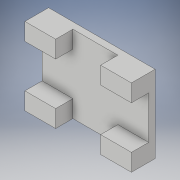
# Autodesk Inventor part: Temporary Guide
Saved by Autodesk Inventor 2018 (Build 220112000, 112)
## iProperties
Created: 2019-01-11
Part Number: Temporary Guide
Material: Generic
Document SubType Name: Modeling
Designer: s-2512711
Density: 1 g/cm^3
Appearance: Default
Author: s-2512711
Autodesk Inventor part; units mm, degrees
ref_plane "YZ Plane" through (0, 0, 0) normal (1, 0, 0) x (0, 1, 0)
ref_plane "XZ Plane" through (0, 0, 0) normal (0, 1, 0) x (-1, 0, 0)
ref_plane "XY Plane" through (0, 0, 0) normal (0, 0, 1) x (1, 0, 0)
sketch "Sketch1" plane through (0, 0, 0) normal (0, 0, 1) x (1, 0, 0)
  line L0 (0, 0) -> (100.33, 0)
  line L1 (100.33, 0) -> (100.33, 72.898)
  line L2 (100.33, 72.898) -> (0, 72.898)
  line L3 (0, 72.898) -> (0, 0)
  dimension "d0" = 100.33
  dimension "d1" = 72.898
  constraints: 8 end point, 2 parallel, 1 horizontal, 1 perpendicular
  measures "d0" distance of L2.end L1.end
  measures "d1" distance of L1.end L0.end
extrude "Extrusion1" add sketch "Sketch1" along normal blind 6.096
sketch "Sketch2" plane through (0, 0, 6.096) normal (0, 0, 1) x (1, 0, 0)
  line L0 (100.33, 72.898) -> (0, 72.898) projected
  line L1 (0, 72.898) -> (28.956, 72.898)
  line L2 (28.956, 72.898) -> (28.956, 56.642)
  line L3 (28.956, 56.642) -> (0, 56.642)
  line L4 (0, 56.642) -> (0, 72.898)
  line L5 (50.165, 72.898) -> (50.165, 0) construction
  line L6 (0, 0) -> (100.33, 0) construction
  line L7 (100.33, 0) -> (100.33, 72.898) construction
  line L8 (100.33, 36.449) -> (0, 36.449) construction
  line L9 (100.33, 72.898) -> (71.374, 72.898)
  line L10 (71.374, 72.898) -> (71.374, 56.642)
  line L11 (71.374, 56.642) -> (100.33, 56.642)
  line L12 (100.33, 56.642) -> (100.33, 72.898)
  line L13 (0, 0) -> (28.956, 0)
  line L14 (28.956, 0) -> (28.956, 16.256)
  line L15 (28.956, 16.256) -> (0, 16.256)
  line L16 (0, 16.256) -> (0, 0)
  line L17 (100.33, 72.898) -> (100.33, 0) construction
  line L18 (100.33, 0) -> (71.374, 0)
  line L19 (71.374, 0) -> (71.374, 16.256)
  line L20 (71.374, 16.256) -> (100.33, 16.256)
  line L21 (100.33, 16.256) -> (100.33, 0)
  dimension "d4" = 28.956
  dimension "d5" = 16.256
  constraints: 38 end point, 11 symmetric about line, 3 midpoint, 2 horizontal, 2 parallel, 1 perpendicular
  measures "d4" distance of L2.end L3.end
  measures "d5" distance of L1.end L2.end
extrude "Extrusion2" add sketch "Sketch2" along normal blind 16.256
body "Solid1"
